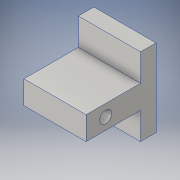
# Autodesk Inventor part: Support For Arms
Saved by Autodesk Inventor 2016 (Build 200138000, 138)
## iProperties
Created: 2015-07-13
Part Number: Support For Arms
Material: Aluminum 6061
Document SubType Name: Modeling
Designer: steele
Density: 2.7 g/cm^3
Appearance: Aluminum - Flat
Author: steele
Autodesk Inventor part; units mm, degrees
ref_plane "YZ Plane" through (0, 0, 0) normal (1, 0, 0) x (0, 1, 0)
ref_plane "XZ Plane" through (0, 0, 0) normal (0, 1, 0) x (-1, 0, 0)
ref_plane "XY Plane" through (0, 0, 0) normal (0, 0, 1) x (1, 0, 0)
sketch "Sketch1" plane through (0, 0, 0) normal (0, 0, 1) x (1, 0, 0)
  line L0 (-25.4, -31.75) -> (25.4, -31.75)
  line L1 (25.4, -31.75) -> (25.4, 31.75)
  line L2 (25.4, 31.75) -> (-25.4, 31.75)
  line L3 (-25.4, 31.75) -> (-25.4, -31.75)
  line L4 (-25.4, -31.75) -> (25.4, 31.75) construction
  line L5 (25.4, -31.75) -> (-25.4, 31.75) construction
  point P0 (0, 0)
  dimension "Back_Height" = 63.5
  dimension "Back_Width" = 50.8
  constraints: 12 end point, 2 midpoint, 2 parallel, 1 horizontal, 1 perpendicular
  measures "Back_Height" distance of L0.end L1.end
  measures "Back_Width" distance of L1.end L2.end
extrude "Extrusion1" add sketch "Sketch1" against normal blind 12.7
sketch "Sketch3" plane through (0, 0, 0) normal (0, 0, 1) x (1, 0, 0)
  line L0 (-25.4, -9.525) -> (25.4, -9.525)
  line L1 (25.4, -9.525) -> (25.4, 9.525)
  line L2 (25.4, 9.525) -> (-25.4, 9.525)
  line L3 (-25.4, 9.525) -> (-25.4, -9.525)
  line L4 (-25.4, -9.525) -> (25.4, 9.525) construction
  line L5 (25.4, -9.525) -> (-25.4, 9.525) construction
  line L6 (25.4, 31.75) -> (-25.4, 31.75) projected
  point P0 (0, 0)
  dimension "Channel_Width" = 19.05
  constraints: 12 end point, 3 parallel, 2 midpoint, 1 perpendicular
  measures "Channel_Width" distance of L1.end L0.end
extrude "Extrusion3" add sketch "Sketch3" along normal blind 44.45
sketch "Sketch5" plane through (-25.4, -9.525, 0) normal (-1, 0, 0) x (0, 0, 1)
  line L0 (0, 9.525) -> (44.45, 9.525) construction
  line L1 (44.45, 19.05) -> (44.45, 0) construction
  line L2 (0, 0) -> (44.45, 0) construction
  line L3 (28.575, 0) -> (28.575, 19.05) construction
  line L4 (0, 19.05) -> (44.45, 19.05) construction
  circle A0 centre (28.575, 9.525) radius 1.27
  dimension "d21" = 28.575
  dimension "d22" = 2.54
  constraints: 4 end point, 2 midpoint, 2 point on line, 1 centre point, 1 perpendicular
  measures "d21" distance from line of L3 L0.start
  measures "d22" diameter of A0
extrude "Extrusion4" cut sketch "Sketch5" against normal through all
hole "Hole4" at (-25.4, 0, 28.575) direction (1, 0, 0) diameter 9.7282 end through all thread size "7/16-20 UNF" class "2B" standard "ANSI Unified Screw Threads"
body "Solid1"
